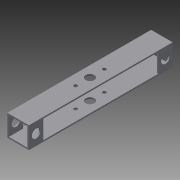
# Autodesk Inventor part: encoder_wheel_support
Saved by Autodesk Inventor 2014 SP1 (Build 180222100, 222)
## iProperties
Created: 2014-09-21
Part Number: encoder_wheel_support
Material: Générique
Document SubType Name: Modeling
Designer: astralien3000
Density: 1 g/cm^3
Appearance: Par défaut
d0: 15,000 mm
d1: 15,000 mm
d2: 7,500 mm
d3: 7,500 mm
d4: 100,000 mm
d5: 0,00 deg
d6: 1,000 mm
d7: 1,000 mm
d8: 1,000 mm
d9: 1,000 mm
d11: 0,00 deg
d12: 80,000 mm
d13: 1,000 mm
d14: 1,000 mm
d16: 50,000 mm
d18: 0,00 deg
d19: 6,000 mm
d21: 0,00 deg
d22: 6,000 mm
d24: 50,000 mm
d25: 7,500 mm
d26: 10,000 mm
d27: 2,500 mm
d29: 0,00 deg
d15: 100,000 mm
d23: 100,000 mm
Author: astralien3000
Autodesk Inventor part; units mm, degrees
ref_plane "YZ Plane" through (0, 0, 0) normal (1, 0, 0) x (0, 1, 0)
ref_plane "XZ Plane" through (0, 0, 0) normal (0, 1, 0) x (-1, 0, 0)
ref_plane "XY Plane" through (0, 0, 0) normal (0, 0, 1) x (1, 0, 0)
sketch "Esquisse1" plane through (0, 0, 0) normal (0, 1, 0) x (-1, 0, 0)
  line L0 (-7.5, 7.5) -> (7.5, 7.5)
  line L1 (7.5, 7.5) -> (7.5, -7.5)
  line L2 (7.5, -7.5) -> (-7.5, -7.5)
  line L3 (-7.5, -7.5) -> (-7.5, 7.5)
  point P0 (0, 0)
  dimension "d0" = 15
  dimension "d1" = 15
  dimension "d2" = 7.5
  dimension "d3" = 7.5
  constraints: 8 end point, 2 parallel, 1 horizontal, 1 perpendicular
  measures "d0" distance of L0.start L0.end
  measures "d1" distance of L0.end L1.end
  measures "d2" distance from line of L0 point (0, 0)
  measures "d3" distance from line of L3 point (0, 0)
extrude "Extrusion1" add sketch "Esquisse1" along normal blind 100
sketch "Esquisse2" plane through (0, 100, 0) normal (0, 1, 0) x (1, 0, 0)
  line L0 (-7.5, -7.5) -> (7.5, -7.5) projected
  line L1 (7.5, -7.5) -> (7.5, 7.5) projected
  line L2 (7.5, 7.5) -> (-7.5, 7.5) projected
  line L3 (-7.5, 7.5) -> (-7.5, -7.5) projected
  line L4 (-6.5, 6.5) -> (6.5, 6.5)
  line L5 (6.5, 6.5) -> (6.5, -6.5)
  line L6 (6.5, -6.5) -> (-6.5, -6.5)
  line L7 (-6.5, -6.5) -> (-6.5, 6.5)
  point P0 (0, 0)
  dimension "d6" = 1
  dimension "d7" = 1
  dimension "d8" = 1
  dimension "d9" = 1
  constraints: 8 end point, 2 parallel, 1 horizontal, 1 perpendicular
  measures "d6" distance between parallel lines of L1 L5
  measures "d7" distance between parallel lines of L2 L4
  measures "d8" distance between parallel lines of L3 L7
  measures "d9" distance between parallel lines of L0 L6
extrude "Extrusion2" cut sketch "Esquisse2" against normal through all contours L4 L5 L6 L7
sketch "Esquisse3" plane through (7.5, 0, 7.5) normal (1, 0, 0) x (0, 0, -1)
  line L0 (15, 0) -> (0, 0) projected
  line L1 (15, 0) -> (15, 100) projected
  line L2 (0, 0) -> (0, 100) projected
  line L3 (1, 90) -> (14, 90)
  line L4 (14, 90) -> (14, 10)
  line L5 (14, 10) -> (1, 10)
  line L6 (1, 10) -> (1, 90)
  line L7 (1, 50) -> (14, 50) construction
  point P0 (7.5, 0)
  dimension "d12" = 80
  dimension "d13" = 1
  dimension "d14" = 1
  dimension "d15" = 100
  dimension "d16" = 50
  constraints: 10 end point, 2 midpoint, 2 parallel, 1 horizontal, 1 perpendicular
  measures "d12" distance of L5.end L3.start
  measures "d13" distance between parallel lines of L1 L4
  measures "d14" distance between parallel lines of L2 L6
  measures "d15" distance of L0.start L1.end
  measures "d16" distance between parallel lines of L0 L7
extrude "Extrusion3" cut sketch "Esquisse3" against normal through all
sketch "Esquisse4" plane through (7.5, 0, 7.5) normal (1, 0, 0) x (0, 0, -1)
  line L0 (1, 10) -> (1, 90) projected
  line L1 (1, 90) -> (14, 90) projected
  line L2 (14, 90) -> (14, 10) projected
  line L3 (15, 0) -> (15, 100) projected
  line L4 (0, 0) -> (0, 100) projected
  line L5 (0, 90) -> (15, 90) construction
  line L6 (0, 90) -> (15, 100) construction
  line L7 (0, 100) -> (15, 90) construction
  circle A0 centre (7.5, 95) radius 3
  line L8 (1, 50) -> (14, 50) construction
  circle A1 centre (7.5, 5) radius 3
  point P0 (7.5, 0)
  dimension "d19" = 6
  constraints: 8 end point, 3 midpoint, 2 centre point, 2 point on line, 1 collinear, 1 perpendicular, 1 other
  measures "d19" diameter of A0
extrude "Extrusion4" cut sketch "Esquisse4" against normal through all
sketch "Esquisse5" plane through (7.5, 0, -7.5) normal (0, 0, -1) x (-1, 0, 0)
  line L0 (15, 0) -> (0, 0) projected
  line L1 (0, 100) -> (15, 100) projected
  line L2 (0, 0) -> (0, 100) projected
  circle A0 centre (7.5, 50) radius 3
  circle A1 centre (7.5, 40) radius 1.25
  circle A2 centre (7.5, 60) radius 1.25
  line L3 (7.5, 50) -> (0, 50) construction
  line L4 (7.5, 50) -> (7.5, 100) construction
  point P0 (7.5, 0)
  dimension "d22" = 6
  dimension "d23" = 100
  dimension "d24" = 50
  dimension "d25" = 7.5
  dimension "d26" = 10
  dimension "d27" = 2.5
  constraints: 4 end point, 3 centre point, 2 midpoint, 1 point on line, 1 other
  measures "d22" diameter of A0
  measures "d23" distance of L0.start L1.end
  measures "d24" distance from line of L0 L3.start
  measures "d25" distance from line of L2 L3.start
  measures "d26" distance of A2.centre L3.start
  measures "d27" diameter of A2
extrude "Extrusion5" cut sketch "Esquisse5" against normal through all
equation "\"d2\" = 0.5 * d1"
equation "\"d3\" = d2"
equation "\"d16\" = 0.5 * d15"
